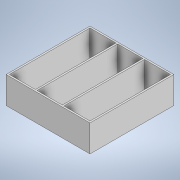
# Autodesk Inventor part: BeadCompartments_4
Saved by Autodesk Inventor 2020 (Build 240168000, 168)
## iProperties
Created: 2022-01-22
Part Number: BeadCompartments_4
Material: Generic
Document SubType Name: Modeling
Designer: danie
Density: 1 g/cm^3
Appearance: Default
Author: danie
Autodesk Inventor part; units mm, degrees
ref_plane "YZ Plane" through (0, 0, 0) normal (1, 0, 0) x (0, 1, 0)
ref_plane "XZ Plane" through (0, 0, 0) normal (0, 1, 0) x (-1, 0, 0)
ref_plane "XY Plane" through (0, 0, 0) normal (0, 0, 1) x (1, 0, 0)
sketch "Sketch1" plane through (0, 0, 0) normal (0, 1, 0) x (-1, 0, 0)
  line L0 (0, 0) -> (-152.4, 0)
  line L1 (-152.4, 0) -> (-152.4, -152.4)
  line L2 (-152.4, -152.4) -> (0, -152.4)
  line L3 (0, -152.4) -> (0, 0)
  line L4 (3.175, 3.175) -> (-155.575, 3.175)
  line L5 (-155.575, 3.175) -> (-155.575, -155.575)
  line L6 (-155.575, -155.575) -> (3.175, -155.575)
  line L7 (3.175, -155.575) -> (3.175, 3.175)
  line L8 (0, 0) -> (-50.8, 0) construction
  line L9 (-50.8, 0) -> (-50.8, -152.4) construction
  line L10 (-50.8, 0) -> (-101.6, 0) construction
  line L11 (-101.6, 0) -> (-101.6, -152.4) construction
  line L12 (-50.8, -41.1467) -> (-49.2125, -41.1467) construction
  line L13 (-50.8, -63.2221) -> (-52.3875, -63.2221) construction
  line L14 (-52.3875, -63.2221) -> (-52.3875, -152.4)
  line L15 (-52.3875, -63.2221) -> (-52.3875, 0)
  line L16 (-49.2125, -41.1467) -> (-49.2125, 0)
  line L17 (-49.2125, -41.1467) -> (-49.2125, -152.4)
  line L18 (-101.6, -10.1231) -> (-100.0125, -10.1231) construction
  line L19 (-101.6, -10.1231) -> (-103.1875, -10.1231) construction
  line L20 (-100.0125, -10.1231) -> (-100.0125, 0)
  line L21 (-103.1875, -10.1231) -> (-103.1875, 0)
  line L22 (-103.1875, -10.1231) -> (-103.1875, -152.4)
  line L23 (-100.0125, -10.1231) -> (-100.0125, -152.4)
  dimension "d0" = 152.4
  dimension "d1" = 152.4
  dimension "d2" = 3.175
  dimension "d3" = 50.8
  dimension "d4" = 50.8
  dimension "d5" = 1.5875
  dimension "d6" = 1.5875
  dimension "d7" = 1.5875
  dimension "d8" = 1.5875
  constraints: 48 end point, 18 point on line, 8 perpendicular, 4 horizontal, 4 parallel, 2 vertical, 3 other
  measures "d0" distance of L2.end L1.end
  measures "d1" distance of L1.end L0.end
  measures "d2" distance between parallel lines of L3 L7
  measures "d3" distance of L0.start L8.end
  measures "d4" distance of L8.end L10.end
  measures "d5" distance of L12.start L12.end
  measures "d6" distance of L13.start L13.end
  measures "d7" distance of L18.start L18.end
  measures "d8" distance of L18.start L19.end
extrude "Extrusion1" add sketch "Sketch1" against normal blind 50.8 contours L16 L17 L2 L14 L15 L0 | L20 L23 L2 L22 L21 L0 | L7 L6 L5 L4
body "Solid1"
